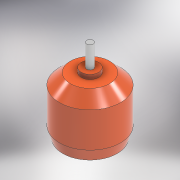
# Autodesk Inventor part: Motor
Saved by Autodesk Inventor 2021.4 (Build 254397000, 397)
## iProperties
Created: 2022-12-11
Part Number: Motor
Material: Genérico
Document SubType Name: Modeling
Designer: crist
Density: 1 g/cm^3
Appearance: Valor por defecto
Author: crist
Autodesk Inventor part; units mm, degrees
ref_plane "YZ Plane" through (0, 0, 0) normal (1, 0, 0) x (0, 1, 0)
ref_plane "XZ Plane" through (0, 0, 0) normal (0, 1, 0) x (-1, 0, 0)
ref_plane "XY Plane" through (0, 0, 0) normal (0, 0, 1) x (1, 0, 0)
sketch "Boceto1" plane through (0, 0, 0) normal (0, 1, 0) x (-1, 0, 0)
  circle A0 centre (0, 0) radius 14
  dimension "d0" = 28
  constraints: 1 centre point, 1 coincident
  measures "d0" diameter of A0
extrude "Extrusión1" add sketch "Boceto1" along normal blind 26
sketch "Boceto2" plane through (0, 26, 0) normal (0, 1, 0) x (1, 0, 0)
  circle A0 centre (0, 0) radius 4
  dimension "d3" = 8
  constraints: 1 centre point, 1 coincident
  measures "d3" diameter of A0
extrude "Extrusión2" add sketch "Boceto2" along normal blind 2
sketch "Boceto3" plane through (0, 28, 0) normal (0, 1, 0) x (1, 0, 0)
  circle A0 centre (0, 0) radius 1.5
  dimension "d6" = 3
  constraints: 1 centre point, 1 coincident
  measures "d6" diameter of A0
extrude "Extrusión3" add sketch "Boceto3" along normal blind 10
sketch "Boceto4" plane through (0, 0, 0) normal (1, 0, 0) x (0, 1, 0)
  line L0 (26, -14) -> (26, 14) projected
  line L1 (26, 14) -> (26, 9)
  line L2 (0, 14) -> (26, 14) projected
  line L3 (21, 14) -> (26, 9)
  line L4 (26, 14) -> (21, 14)
  line L5 (29.3126, 0) -> (24.3126, 0)
  line L6 (0, -14) -> (0, 14) projected
  line L7 (0, 14) -> (0, 12.5)
  line L8 (0, 14) -> (5, 14)
  line L9 (0, 14) -> (26, 14) projected
  line L10 (5, 14) -> (0, 12.5)
  point P0 (0, 0)
  dimension "d9" = 5
  dimension "d11" = 5
  dimension "d13" = 1.5
  dimension "d14" = 5
  constraints: 14 end point, 4 point on line, 1 horizontal
  measures "d9" distance of L0.end L1.end
  measures "d11" distance of L5.start L5.end
  measures "d13" distance of L2.start L7.end
  measures "d14" distance of L2.start L8.end
revolve "Revolución1" cut sketch "Boceto4" angle 360 about axis through (0, 29.3126, 0) along (0, -1, 0)
